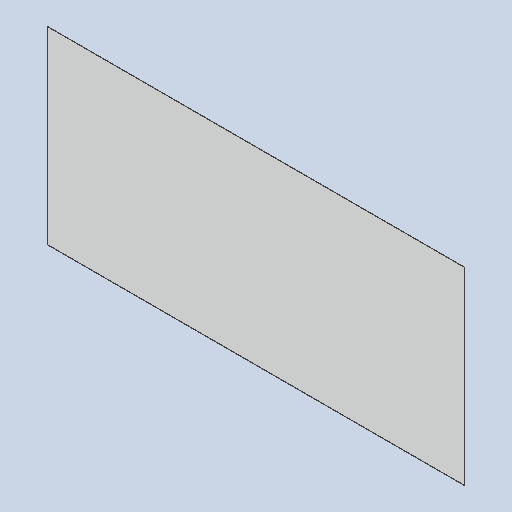
# Autodesk Inventor part: acrilicoFixo
Saved by Autodesk Inventor 2023 (Build 270158000, 158)
## iProperties
Created: 2022-08-29
Part Number: acrilicoFixo
Material: Generic
Document SubType Name: Modeling
Designer: cvss2
Density: 1 g/cm^3
Appearance: Default
Author: cvss2
Autodesk Inventor part; units mm, degrees
ref_plane "YZ Plane" through (0, 0, 0) normal (1, 0, 0) x (0, 1, 0)
ref_plane "XZ Plane" through (0, 0, 0) normal (0, 1, 0) x (-1, 0, 0)
ref_plane "XY Plane" through (0, 0, 0) normal (0, 0, 1) x (1, 0, 0)
sketch "Sketch1" plane through (0, 0, 0) normal (0, 0, 1) x (1, 0, 0)
  line L0 (0, 0) -> (-2560, 0)
  line L1 (-2560, 0) -> (-2560, 1160)
  line L2 (-2560, 1160) -> (0, 1160)
  line L3 (0, 1160) -> (0, 0)
  dimension "d0" = 2560
  dimension "d1" = 1160
  constraints: 8 end point, 2 parallel, 1 horizontal, 1 perpendicular
  measures "d0" distance of L1.end L2.end
  measures "d1" distance of L0.end L1.end
extrude "Extrusion1" add sketch "Sketch1" against normal blind 2
body "Solid1"
